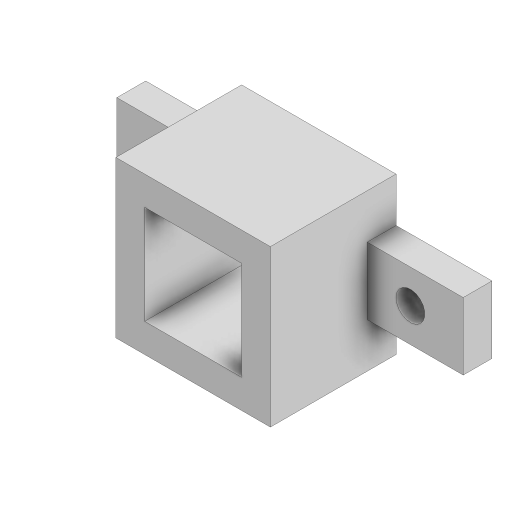
# Autodesk Inventor part: adapter_for_magnet
Saved by Autodesk Inventor 2024 (Build 280153000, 153)
## iProperties
Created: 2023-11-12
Part Number: adapter_for_magnet
Material: 一般
Document SubType Name: Modeling
Designer: moonshot
Density: 1 g/cm^3
Appearance: 既定
Author: moonshot
Autodesk Inventor part; units mm, degrees
ref_plane "YZ Plane" through (0, 0, 0) normal (1, 0, 0) x (0, 1, 0)
ref_plane "XZ Plane" through (0, 0, 0) normal (0, 1, 0) x (-1, 0, 0)
ref_plane "XY Plane" through (0, 0, 0) normal (0, 0, 1) x (1, 0, 0)
sketch "スケッチ1" plane through (0, 0, 0) normal (0, 0, 1) x (1, 0, 0)
  line L0 (-5.05, 5.1477) -> (5.05, 5.1477)
  line L1 (5.05, 5.1477) -> (5.05, -5.1477)
  line L2 (5.05, -5.1477) -> (-5.05, -5.1477)
  line L3 (-5.05, -5.1477) -> (-5.05, 5.1477)
  line L4 (0, -11.4068) -> (0, 11.4068) projected
  line L5 (-11.27, 0) -> (11.27, 0) projected
  line L6 (8.05, 8.1477) -> (-8.05, 8.1477)
  line L7 (-8.05, 8.1477) -> (-8.05, -8.1477)
  line L8 (-8.05, -8.1477) -> (8.05, -8.1477)
  line L9 (8.05, -8.1477) -> (8.05, 8.1477)
  point P0 (0, 0)
  dimension "d0" = 10.1
  dimension "d1" = 3
  constraints: 16 end point, 4 parallel, 2 perpendicular, 1 horizontal, 5 other
  measures "d0" distance of L0.start L0.end
  measures "d1" distance between parallel lines of L0 L6
extrude "押し出し1" add sketch "スケッチ1" along normal mid plane 10.1 contours L3 L5 L7 L6 L4 L0 | L4 L6 L9 L5 L1 L0 | L3 L2 L4 L8 L7 L5 | L5 L9 L8 L4 L2 L1
sketch "スケッチ2" plane through (0, 0, -5.05) normal (0, 0, -1) x (-1, 0, 0)
  line L0 (-8.05, -8.1477) -> (-8.05, 8.1477) projected
  line L1 (-8.05, 3.5) -> (-18.05, 3.5)
  line L2 (-18.05, 3.5) -> (-18.05, -3.5)
  line L3 (-18.05, -3.5) -> (-8.05, -3.5)
  line L4 (8.05, 8.1477) -> (-8.05, 8.1477) projected
  line L5 (-8.05, -8.1477) -> (8.05, -8.1477) projected
  line L6 (8.05, -8.1477) -> (8.05, 8.1477) projected
  line L7 (8.05, 8.1477) -> (-8.05, 8.1477) projected
  line L8 (-8.05, 8.1477) -> (-8.05, -8.1477) projected
  line L9 (5.05, 5.1477) -> (5.05, -5.1477) projected
  line L10 (5.05, -5.1477) -> (-5.05, -5.1477) projected
  line L11 (-5.05, -5.1477) -> (-5.05, 5.1477) projected
  line L12 (-5.05, 5.1477) -> (5.05, 5.1477) projected
  line L13 (-8.05, 3.5) -> (-8.05, 8.1477)
  line L14 (-8.05, 8.1477) -> (8.05, 8.1477) projected
  line L15 (-8.05, 8.1477) -> (8.05, 8.1477)
  line L16 (8.05, 3.5) -> (18.05, 3.5)
  line L17 (18.05, 3.5) -> (18.05, -3.5)
  line L18 (18.05, -3.5) -> (8.05, -3.5)
  line L19 (8.05, 8.1477) -> (8.05, 3.5)
  line L20 (8.05, 8.1477) -> (8.05, -8.1477) projected
  line L21 (8.05, -3.5) -> (8.05, -8.1477)
  line L22 (8.05, -8.1477) -> (-8.05, -8.1477)
  line L23 (-8.05, -8.1477) -> (-8.05, -3.5)
  line L24 (22.47, 0) -> (-22.47, 0) projected
  line L25 (0, -11.4068) -> (0, 11.4068) projected
  circle A0 centre (-12.55, 0) radius 1.5
  circle A1 centre (12.55, 0) radius 1.5
  point P0 (0, 0)
  dimension "d4" = 3
  dimension "d5" = 3
  dimension "d8" = 2
  dimension "d11" = 4
  dimension "d12" = 4.5
  constraints: 24 end point, 6 point on line, 5 collinear, 5 perpendicular, 2 centre point, 2 horizontal, 1 symmetric about line, 1 vertical, 3 other
  measures "d4" diameter of A0
  measures "d5" diameter of A1
  measures "d8" distance edge to line of A0 L1
  measures "d11" distance edge to line of A0 L2
  measures "d12" distance from line of A0.centre L0
extrude "押し出し2" add sketch "スケッチ2" along normal blind 3 contours L0 L24 L11 L10 L25 L5 | L3 L2 L24 A0 L0 | L25 L10 L9 L24 L6 L5 | L24 A0 L2 L1 L0 | L0 L4 L25 L12 L11 L24 | L25 L24 L9 L10 | L10 L11 L24 L25 | L11 L12 L25 L24 | L6 L24 A1 L17 L18 | L25 L12 L9 L24 | L24 L9 L12 L25 L4 L6 | L6 L16 L17 L24 A1
